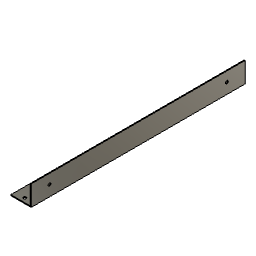
Bottom Angle 1.5 inch 400 mm Left v6 (Autodesk Fusion 360 design; units mm, degrees)
Autodesk Fusion 360 part; units mm, degrees
sketch "Sketch1" plane through (0, 0, 0) normal (0, 1, 0) x (1, 0, 0)
  line L0 (-38.1, 0) -> (0, 0)
  line L1 (0, 0) -> (0, -38.1)
  line L2 (-38.1, -1.5875) -> (-1.5875, -1.5875)
  line L3 (-1.5875, -1.5875) -> (-1.5875, -38.1)
  line L4 (-1.5875, -38.1) -> (0, -38.1)
  line L5 (-38.1, -1.5875) -> (-38.1, 0)
  dimension "d5" = 38.1
  dimension "d6" = 1.5875
  constraint horizontal L0
  constraint perpendicular L0 L1
  constraint coincident L0.end L1.start
  constraint equal L0 L1
  constraint perpendicular L1 L4
  constraint perpendicular L0 L5
  measures "d5" distance of L0.end L1.end
extrude "Extrude1" add sketch "Sketch1" along normal blind 400
sketch "Sketch2" plane through (0, 0, 1.5875) normal (0, 0, 1) x (-1, 0, 0)
  line L0 (38.1, 0) -> (1.5875, 0)
  line L1 (1.5875, 0) -> (1.5875, -400)
  line L2 (1.5875, -400) -> (38.1, -400)
  line L3 (38.1, -400) -> (38.1, 0)
  circle A0 centre (10, -392) radius 3.6564
  line L4 (0, 0) -> (0, -400)
  circle A1 centre (20, -8) radius 4.5897
  dimension "d7" = 8
  dimension "d9" = 10
  dimension "d10" = 8
  dimension "d11" = 20
  measures "d7" distance of L2 A0.centre
  measures "d9" distance of A0.centre L4
  measures "d10" distance of L0 A1.centre
  measures "d11" distance of L4 A1.centre
hole "Hole1" at (-20, 8, 1.5875) at (-10, 392, 1.5875) direction (0, 0, -1) diameter 5.5 depth 7 tip angle 118
sketch "Sketch3" plane through (-1.5875, 0, 0) normal (-1, 0, 0) x (0, -1, 0)
  line L0 (0, 1.5875) -> (0, 38.1)
  line L1 (0, 38.1) -> (-400, 38.1)
  line L2 (-400, 38.1) -> (-400, 1.5875)
  line L3 (-400, 1.5875) -> (0, 1.5875)
  circle A0 centre (-365.715, 19.8375) radius 7.0711
  circle A1 centre (-34.285, 19.8375) radius 7.0711
  dimension "d15" = 34.285
  dimension "d16" = 34.285
  dimension "d17" = 18.25
  constraint equal A0 A1
  constraint horizontal A0.centre A1.centre
  measures "d15" distance of L2 A0.centre
  measures "d16" distance of L0 A1.centre
  measures "d17" distance of L3 A0.centre
hole "Hole2" at (-1.5875, 34.285, 19.8375) at (-1.5875, 365.715, 19.8375) direction (1, 0, 0) diameter 5.5 depth 7 tip angle 118
equation "d15 = 23.175 mm + 11.11 mm"
